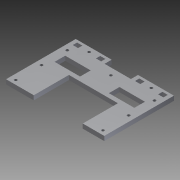
# Autodesk Inventor part: carro x lado motor pieza 1
Saved by Autodesk Inventor 2012 (Build 160160000, 160)
## iProperties
Created: 2014-12-17
Part Number: carro x lado motor pieza 1
Material: Default
Document SubType Name: Modeling
Designer: PRINCIPAL
Density: 1 g/cm^3
Author: PRINCIPAL
Autodesk Inventor part; units mm, degrees
ref_plane "YZ Plane" through (0, 0, 0) normal (1, 0, 0) x (0, 1, 0)
ref_plane "XZ Plane" through (0, 0, 0) normal (0, 1, 0) x (-1, 0, 0)
ref_plane "XY Plane" through (0, 0, 0) normal (0, 0, 1) x (1, 0, 0)
sketch "Boceto1" plane through (0, 0, 0) normal (0, 0, 1) x (1, 0, 0)
  arc A0 (-116.1173, 21.3488) -> (-117.6673, 19.7988) centre (-116.1173, 19.7988) ccw
  arc A1 (-117.6673, 19.7988) -> (-116.1173, 18.2488) centre (-116.1173, 19.7988) ccw
  arc A2 (-116.1173, 18.2488) -> (-114.5673, 19.7988) centre (-116.1173, 19.7988) ccw
  arc A3 (-114.5673, 19.7988) -> (-116.1173, 21.3488) centre (-116.1173, 19.7988) ccw
  arc A4 (-67.1173, 21.3488) -> (-68.6673, 19.7988) centre (-67.1173, 19.7988) ccw
  arc A5 (-68.6673, 19.7988) -> (-67.1173, 18.2488) centre (-67.1173, 19.7988) ccw
  arc A6 (-67.1173, 18.2488) -> (-65.5673, 19.7988) centre (-67.1173, 19.7988) ccw
  arc A7 (-65.5673, 19.7988) -> (-67.1173, 21.3488) centre (-67.1173, 19.7988) ccw
  arc A8 (-18.1173, 21.3488) -> (-19.6673, 19.7988) centre (-18.1173, 19.7988) ccw
  arc A9 (-19.6673, 19.7988) -> (-18.1173, 18.2488) centre (-18.1173, 19.7988) ccw
  arc A10 (-18.1173, 18.2488) -> (-16.5673, 19.7988) centre (-18.1173, 19.7988) ccw
  arc A11 (-16.5673, 19.7988) -> (-18.1173, 21.3488) centre (-18.1173, 19.7988) ccw
  arc A12 (-18.1173, -7.6512) -> (-19.6673, -9.2012) centre (-18.1173, -9.2012) ccw
  arc A13 (-19.6673, -9.2012) -> (-18.1173, -10.7512) centre (-18.1173, -9.2012) ccw
  arc A14 (-18.1173, -10.7512) -> (-16.5673, -9.2012) centre (-18.1173, -9.2012) ccw
  arc A15 (-16.5673, -9.2012) -> (-18.1173, -7.6512) centre (-18.1173, -9.2012) ccw
  arc A16 (-116.1173, -7.6512) -> (-117.6673, -9.2012) centre (-116.1173, -9.2012) ccw
  arc A17 (-117.6673, -9.2012) -> (-116.1173, -10.7512) centre (-116.1173, -9.2012) ccw
  arc A18 (-116.1173, -10.7512) -> (-114.5673, -9.2012) centre (-116.1173, -9.2012) ccw
  arc A19 (-114.5673, -9.2012) -> (-116.1173, -7.6512) centre (-116.1173, -9.2012) ccw
  arc A20 (-116.1173, -36.6512) -> (-117.6673, -38.2012) centre (-116.1173, -38.2012) ccw
  arc A21 (-117.6673, -38.2012) -> (-116.1173, -39.7512) centre (-116.1173, -38.2012) ccw
  arc A22 (-116.1173, -39.7512) -> (-114.5673, -38.2012) centre (-116.1173, -38.2012) ccw
  arc A23 (-114.5673, -38.2012) -> (-116.1173, -36.6512) centre (-116.1173, -38.2012) ccw
  arc A24 (-18.1173, -36.6512) -> (-19.6673, -38.2012) centre (-18.1173, -38.2012) ccw
  arc A25 (-19.6673, -38.2012) -> (-18.1173, -39.7512) centre (-18.1173, -38.2012) ccw
  arc A26 (-18.1173, -39.7512) -> (-16.5673, -38.2012) centre (-18.1173, -38.2012) ccw
  arc A27 (-16.5673, -38.2012) -> (-18.1173, -36.6512) centre (-18.1173, -38.2012) ccw
  arc A28 (-102.1173, 31.8488) -> (-103.6673, 30.2988) centre (-102.1173, 30.2988) ccw
  arc A29 (-103.6673, 30.2988) -> (-102.1173, 28.7488) centre (-102.1173, 30.2988) ccw
  arc A30 (-102.1173, 28.7488) -> (-100.5673, 30.2988) centre (-102.1173, 30.2988) ccw
  arc A31 (-100.5673, 30.2988) -> (-102.1173, 31.8488) centre (-102.1173, 30.2988) ccw
  arc A32 (-32.1173, 31.8488) -> (-33.6673, 30.2988) centre (-32.1173, 30.2988) ccw
  arc A33 (-33.6673, 30.2988) -> (-32.1173, 28.7488) centre (-32.1173, 30.2988) ccw
  arc A34 (-32.1173, 28.7488) -> (-30.5673, 30.2988) centre (-32.1173, 30.2988) ccw
  arc A35 (-30.5673, 30.2988) -> (-32.1173, 31.8488) centre (-32.1173, 30.2988) ccw
  line L0 (-22.3173, 1.3488) -> (-22.3173, 13.2488)
  line L1 (-22.3173, 13.2488) -> (-50.9173, 13.2488)
  line L2 (-50.9173, 13.2488) -> (-50.9173, 1.3488)
  line L3 (-50.9173, 1.3488) -> (-22.3173, 1.3488)
  line L4 (-83.3173, 1.3488) -> (-83.3173, 13.2488)
  line L5 (-83.3173, 13.2488) -> (-111.9173, 13.2488)
  line L6 (-111.9173, 13.2488) -> (-111.9173, 1.3488)
  line L7 (-111.9173, 1.3488) -> (-83.3173, 1.3488)
  line L8 (-86.2223, 27.9117) -> (-86.2223, 32.6859)
  line L9 (-86.2223, 32.6859) -> (-92.0123, 32.6859)
  line L10 (-92.0123, 32.6859) -> (-92.0123, 27.9117)
  line L11 (-92.0123, 27.9117) -> (-86.2223, 27.9117)
  line L12 (-112.1673, 27.8663) -> (-112.1673, 32.7313)
  line L13 (-112.1673, 32.7313) -> (-118.0673, 32.7313)
  line L14 (-118.0673, 32.7313) -> (-118.0673, 27.8663)
  line L15 (-118.0673, 27.8663) -> (-112.1673, 27.8663)
  line L16 (-42.1673, 27.8663) -> (-42.1673, 32.7313)
  line L17 (-42.1673, 32.7313) -> (-48.0673, 32.7313)
  line L18 (-48.0673, 32.7313) -> (-48.0673, 27.8663)
  line L19 (-48.0673, 27.8663) -> (-42.1673, 27.8663)
  line L20 (-16.1673, 27.8663) -> (-16.1673, 32.7313)
  line L21 (-16.1673, 32.7313) -> (-22.0673, 32.7313)
  line L22 (-22.0673, 32.7313) -> (-22.0673, 27.8663)
  line L23 (-22.0673, 27.8663) -> (-16.1673, 27.8663)
  line L24 (-36.0566, -42.9012) -> (-36.0566, -3.3934)
  line L25 (-36.0566, -3.3934) -> (-41.3173, -3.3934)
  line L26 (-41.3173, -3.3934) -> (-80.1673, -3.3934)
  line L27 (-80.1673, -3.3934) -> (-91.1173, -3.3934)
  line L28 (-91.1173, -3.3934) -> (-91.1173, -42.9012)
  line L29 (-91.1173, -42.9012) -> (-122.3173, -42.9012)
  line L30 (-122.3173, -42.9012) -> (-122.3173, 35.4988)
  line L31 (-122.3173, 35.4988) -> (-81.9173, 35.4988)
  line L32 (-81.9173, 35.4988) -> (-81.9173, 27.4988)
  line L33 (-81.9173, 27.4988) -> (-52.3173, 27.4988)
  line L34 (-52.3173, 27.4988) -> (-52.3173, 35.4988)
  line L35 (-52.3173, 35.4988) -> (-11.9173, 35.4988)
  line L36 (-11.9173, 35.4988) -> (-11.9173, -42.9012)
  line L37 (-11.9173, -42.9012) -> (-36.0566, -42.9012)
  point P0 (0, 0)
  constraints: 76 end point, 72 point on circle, 36 centre point
extrude "Extrusión1" add sketch "Boceto1" along normal blind 5
